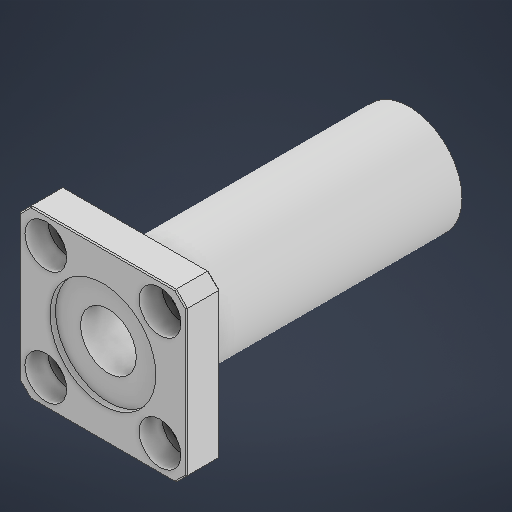
# Autodesk Inventor part: RolamentoLinear10d
Saved by Autodesk Inventor 2025.2 (Build 292293000, 293)
## iProperties
Created: 2025-04-06
Part Number: RolamentoLinear10d
Material: Generic
Document SubType Name: Modeling
Designer: Tiago
Density: 1 g/cm^3
Appearance: Default
Author: Tiago
Autodesk Inventor part; units mm, degrees
ref_plane "YZ Plane" through (0, 0, 0) normal (1, 0, 0) x (0, 1, 0)
ref_plane "XZ Plane" through (0, 0, 0) normal (0, 1, 0) x (-1, 0, 0)
sketch "Sketch1" plane through (0, 0, 0) normal (0, 0, 1) x (1, 0, 0)
  circle A0 centre (0, 0) radius 5
  circle A1 centre (0, 0) radius 9.5
  circle A2 centre (0, 0) radius 8.5
  dimension "d" = 10
  dimension "D" = 19
  dimension "d23" = 17
  constraints: 3 centre point, 3 coincident
  measures "d" diameter of A0
  measures "D" diameter of A1
  measures "d23" diameter of A2
extrude "Extrusion1" add sketch "Sketch1" along normal blind 49 contours A1 | A2
sketch "Sketch2" plane through (0, 0, 49) normal (0, 0, 1) x (1, 0, 0)
  circle A0 centre (0, 0) radius 9.5
  line L0 (-15, -15) -> (15, -15)
  line L1 (15, -15) -> (15, 15)
  line L2 (15, 15) -> (-15, 15)
  line L3 (-15, 15) -> (-15, -15)
  line L4 (-15, -15) -> (15, 15) construction
  line L5 (15, -15) -> (-15, 15) construction
  circle A1 centre (0, 0) radius 14.5 construction
  circle A2 centre (10.253, 10.253) radius 2.25
  circle A3 centre (10.253, 10.253) radius 3.75
  line L6 (-5.4596, 0) -> (5.4596, 0) construction
  line L7 (0, -5.5798) -> (0, 5.5798) construction
  circle A4 centre (10.253, -10.253) radius 2.25
  circle A5 centre (10.253, -10.253) radius 3.75
  circle A6 centre (-10.253, 10.253) radius 2.25
  circle A7 centre (-10.253, 10.253) radius 3.75
  circle A8 centre (-10.253, -10.253) radius 3.75
  circle A9 centre (-10.253, -10.253) radius 2.25
  circle A10 centre (0, 0) radius 5
  point P0 (15, 0)
  point P1 (0, 15)
  point P2 (0, 0)
  point P3 (0, 0)
  dimension "DP" = 29
  dimension "k" = 30
  dimension "d27" = 30
  dimension "X" = 4.5
  dimension "Y" = 7.5
  constraints: 16 end point, 10 centre point, 7 coincident, 6 midpoint, 6 symmetric about line, 2 horizontal, 2 parallel, 1 horizontal alignment, 1 perpendicular, 1 point on line, 1 vertical, 1 vertical alignment, 9 other
  measures "k" distance of L0.end L1.end
  measures "d27" distance of L1.end L2.end
  measures "X" diameter of A2
  measures "Y" diameter of A3
ref_plane "Work Plane1" through (0, 0, 55) normal (0, 0, 1) x (1, 0, 0)
extrude "Extrusion6" cut sketch "Sketch1" along normal blind 1 contours A2
extrude "Extrusion7" add sketch "Sketch2" along normal blind 6 contours L3 L2 L1 L0
chamfer "Chamfer1" distance 2 angle 45 4 edges at (-15, -15, 52) (15, -15, 52) (15, 15, 52) (-15, 15, 52)
extrude "Extrusion8" add sketch "Sketch2" along normal blind 1.9 contours A3 | A5 | A7 | A8
extrude "Extrusion9" add sketch "Sketch2" along normal blind 5 contours A0
chamfer "Chamfer2" distance 0.2 angle 45 16 edges at (0, -15, 55) (-15, 0, 55) (0, 15, 55) (15, 0, 55) (14, -14, 55) (-14, -14, 55) (-14, 14, 55) (14, 14, 55) (-14, -14, 49) (0, -15, 49) (-15, 0, 49) (14, -14, 49) (15, 0, 49) (14, 14, 49) (0, 15, 49) (-14, 14, 49)
equation "\"d27\" = k"
equation "\"d36\" = t - z"
equation "\"z\" = 4.1"
equation "\"t\" = 6"
body "Solid1"
